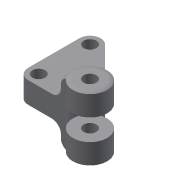
# Autodesk Inventor part: tribar
Saved by Autodesk Inventor 2018 (Build 220112000, 112)
## iProperties
Created: 2018-08-17
Part Number: tribar
Material: Generic
Document SubType Name: Modeling
Designer: Bardo91
Density: 1 g/cm^3
Appearance: Default
Author: Bardo91
Autodesk Inventor part; units mm, degrees
ref_plane "YZ Plane" through (0, 0, 0) normal (1, 0, 0) x (0, 1, 0)
ref_plane "XZ Plane" through (0, 0, 0) normal (0, 1, 0) x (-1, 0, 0)
ref_plane "XY Plane" through (0, 0, 0) normal (0, 0, 1) x (1, 0, 0)
sketch "Sketch1" plane through (0, 0, 0) normal (0, 0, 1) x (1, 0, 0)
  line L0 (0, 0) -> (0, 12)
  line L1 (0, 0) -> (12, 0)
  arc A0 (12, -2.5) -> (13.7678, 1.7678) centre (12, 0) ccw
  arc A1 (-2.5, 0) -> (0, -2.5) centre (0, 0) ccw
  arc A2 (1.7678, 13.7678) -> (-2.5, 12) centre (0, 12) ccw
  line L2 (0, 0) -> (0, -2.5)
  line L3 (0, -2.5) -> (12, -2.5)
  line L4 (0, 12) -> (-2.5, 12)
  line L5 (-2.5, 12) -> (-2.5, 0)
  line L6 (1.7678, 13.7678) -> (13.7678, 1.7678)
  dimension "d14" = 12
  dimension "d15" = 12
  dimension "d16" = 5
  dimension "d17" = 5
  dimension "d18" = 5
  constraints: 14 end point, 6 point on circle, 3 centre point, 3 coincident, 2 perpendicular, 2 vertical, 1 horizontal, 1 parallel
  measures "d14" distance of L0.start L0.end
  measures "d15" distance of L0.start L1.end
  measures "d16" diameter of A0
  measures "d17" diameter of A1
  measures "d18" diameter of A2
extrude "Extrusion1" add sketch "Sketch1" along normal blind 5
sketch "Sketch2" plane through (0, 0, 0) normal (0, 0, -1) x (-1, 0, 0)
  arc A0 (-13.7678, 1.7678) -> (-12, -2.5) centre (-12, 0) ccw projected
  circle A1 centre (-12, 0) radius 4
  point P0 (0, 0)
  dimension "d19" = 8
  constraints: 1 centre point, 1 coincident
  measures "d19" diameter of A1
extrude "Extrusion2" add sketch "Sketch2" along normal blind 5 and the other way blind 10
sketch "Sketch3" plane through (0, 0, 0) normal (0, 0, -1) x (-1, 0, 0)
  circle A0 centre (-12, 0) radius 4 projected
  circle A1 centre (-12, 0) radius 3.5
  point P0 (0, 0)
  dimension "d24" = 7
  constraints: 1 centre point, 1 coincident
  measures "d24" diameter of A1
extrude "Extrusion3" cut sketch "Sketch3" against normal blind 5 contours A0 | A1
sketch "Sketch4" plane through (0, 0, 5) normal (0, 0, 1) x (1, 0, 0)
  circle A0 centre (12, 0) radius 4 projected
  arc A1 (10.7059, 4.8296) -> (7.6699, -2.5) centre (12, 0) ccw
  line L0 (11.5598, 3.9757) -> (1.7678, 13.7678) projected
  line L1 (10.7059, 4.8296) -> (11.5598, 3.9757)
  line L2 (0, -2.5) -> (8.8775, -2.5) projected
  line L3 (8.8775, -2.5) -> (7.6699, -2.5)
  arc A2 (11.5598, 3.9757) -> (8.8775, -2.5) centre (12, 0) ccw
  point P0 (0, 0)
  dimension "d27" = 10
  constraints: 4 end point, 4 point on circle, 2 centre point, 2 coincident, 2 point on line, 1 collinear, 1 concentric
  measures "d27" diameter of A1
extrude "Extrusion4" add sketch "Sketch4" along normal blind 5 and the other way blind 10 contours A0 L2 A1 L0
fillet "Fillet1" radius 2 4 edges at (7.3806, 1.9134, 5) (7.3806, 1.9134, 0) (7.3806, 1.9134, -5) (7.3806, 1.9134, 10)
sketch "Sketch5" plane through (0, 0, 10) normal (0, 0, 1) x (1, 0, 0)
  arc A0 (1.7678, 13.7678) -> (-2.5, 12) centre (0, 12) ccw projected
  circle A1 centre (0, 12) radius 1.5
  circle A2 centre (0, 0) radius 1.5
  arc A3 (8.8775, -2.5) -> (11.5598, 3.9757) centre (12, 0) ccw projected
  circle A4 centre (12, 0) radius 1.5
  dimension "d33" = 3
  dimension "d34" = 3
  dimension "d35" = 3
  constraints: 3 centre point, 3 coincident
  measures "d33" diameter of A1
  measures "d34" diameter of A2
  measures "d35" diameter of A4
extrude "Extrusion5" cut sketch "Sketch5" against normal through all
body "Solid1"
